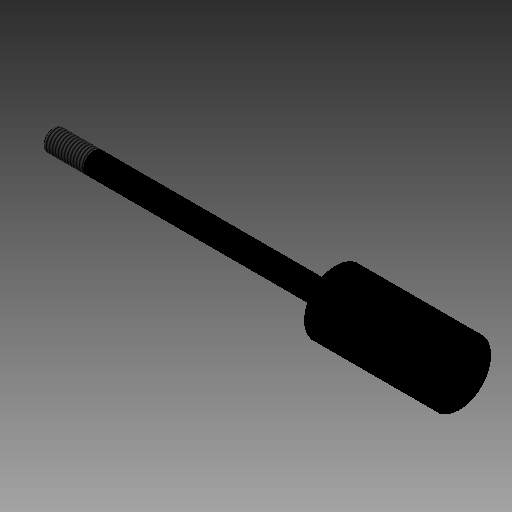
# Autodesk Inventor part: C-0420000_rod
Saved by Autodesk Inventor 2018.3 (Build 223284000, 284)
## iProperties
Category: PARTsolutions
Company: BIMBA
Created: 2019-01-30
Part Number: C-0420000_rod
Material: Generic
Catalog Web Link: www.cadenas.de
Description: Standard Air Cylinder_rod-Original Line - Standard Air Cylinders
Vendor: BIMBA
Document SubType Name: Modeling
Designer: psadmin
Manufacturer: BIMBA
Mass: 13.5965 g
Surface Area: 45.5733 cm^2
Volume: 13.5965 cm^3
Density: 1 g/cm^3
Appearance: PSOLRGB-0-0-0
PSOL_IDENT_0: {$CADENAS_DATA\23d-libs\bimba\bimba\bimba_imperial\bimba_full_line\original_line_cylinders\standard_
PSOL_IDENT_1: air_cylinders\rod.prj},319 {VTYP=3D},{NB=C-0420000_rod},{LINA=C-0420000_rod},{NN=Standard Air Cylind
PSOL_IDENT_2: er_rod},{DATE=21.03.2018 14:31:21},{GEOMDATE=09.11.2017 13:09:15},{VERSION=},{LINEID=50},{WBVAR=STRO
PSOL_IDENT_3: KE,ACTING,MNT,DER,NR,BM,CO,M,EE,EEL,K,Q,Y,F,G,T,B,H,SER,SR,NT,W,E,HL,ST,STP,PRC,PB,COLOR1,FCD,RCD,BC
PSOL_IDENT_4: D},{WBNUMERIC=STROKE,EEL,COLOR1,FCD,RCD,BCD}  {NB=C-0420000_rod},{LINA=C-0420000_rod},{KT=DUMMY},{PN=
PSOL_IDENT_5: C-042000},{DASH=},{BORE=0.75000000},{BOREPN=04},{STROKE=2.000},{STROKEALG=[0.001:50/0.001]},{STROKE1=
PSOL_IDENT_6: 2.000},{ACTING=},{ACTINGALG= '' , 'Single Acting' , 'R' , 'Reverse Single Acting' , 'D' , 'Double Ac
PSOL_IDENT_7: ting' },{ACTINGPN=},{MNT=},{MNTALG= '' , 'Front Nose Mounting' , 'P' , 'Rear Pivot Mounting' , 'BF'
PSOL_IDENT_8: , 'Front Block Mounting' , 'BR' , 'Rear Block Mounting for Vertical Positioning' , 'BFT' , 'Front Bl
PSOL_IDENT_9: ock Trunnion Mounting' , 'BRT' , 'Rear Block Trunnion Mounting' , 'A' , 'Double End Mounting with Br
PSOL_IDENT_10: ackets and Adjustable Stroke' , 'AP' , 'Rear Pivot Mounting with Adjustable Stroke' },{TYPE=C-},{MNT
PSOL_IDENT_11: PN=},{DER=},{DERALG= '' , 'N/A' },{NR=},{NRALG= '' , 'Standard' , 'NR' , 'Non-rotating - Hexagon Rod'
PSOL_IDENT_12: },{NRPN=},{BM=},{BMALG= '' , 'Without Built-in Midget 3-Way Solenoid Operated Valve' , 'LS' , 'With
PSOL_IDENT_13: Built-in Midget 3-Way Solenoid Operated Valve' },{BMPN=},{CO=},{COALG= '' , 'N/A' },{M=},{MALG= '',
PSOL_IDENT_14: 'Without Magnet', 'M', 'With Magnet' },{EE=},{EEL=0},{EEMAX=10},{EEALG= '', 'Without Extra Extensio
PSOL_IDENT_15: n', 'EE', 'With Extra Extension' },{EELALG=0},{EEPN=},{EEPN1=0.000},{K=},{KALG= '' , 'N/A' },{KPN=},
PSOL_IDENT_16: {Q=},{QALG= '' , 'Without Side Ported Rear Head' , 'Q' , 'With Side Ported Rear Head' },{QPN=},{Y=},
PSOL_IDENT_17: {YALG= '' , 'N/A' },{YPN=},{F=},{FALG= '', 'Standard', 'F', 'Molycoated Body' },{FPN=},{G=},{GPN=},{
PSOL_IDENT_18: T=},{TALG= '' , 'Standard' , 'N' , 'Low Temperature' , 'V' , 'High Temperature' },{NPN=},{VPN=},{B=}
PSOL_IDENT_19: ,{BALG= '', 'Without Bumper' , 'B' , 'With Bumper' },{BPN=},{H=},{HALG= '', 'Standard', 'H', 'With H
PSOL_IDENT_20: eavy Springs' },{HPN=},{SER=},{SERALG= '' , 'N/A' },{SR=C},{SRALG= 'C' , 'Carbon Steel Rod' , 'SR' ,
PSOL_IDENT_21: '303 Stainless Steel Rod' , '' , '303 Stainless Steel Rod1' },{SRPN=C},{SRCON=1},{NT=},{NTPN=},{W=}
PSOL_IDENT_22: ,{WALG= '' , 'N/A' },{WPN=},{E=},{EALG= '' , 'Without Special Lube and Seals' , 'E' , 'With Special
PSOL_IDENT_23: Lube and Seals' },{EPN=},{HL=},{HLALG= '' , 'N/A' },{ST=},{STALG= '' , 'Without Switch Track' , 'T'
PSOL_IDENT_24: , 'With Switch Track' },{STP=},{STPALG= '' , 'N/A' },{STPN=},{PRC=},{PRCALG= '' , 'Without Piston Ro
PSOL_IDENT_25: d Clevis' , 'D-166-1' , 'With Piston Rod Clevis' },{PRCPN=},{PB=},{PBALG= '' , 'Without Pivot Bracke
PSOL_IDENT_26: t' , 'D-167' , 'With Pivot Bracket' },{PBPN=},{TLEN=3.9460},{TEXT=0.233333},{SPACE=0.133333},{FRAC=5
PSOL_IDENT_27: .5700},{RGCON=},{RGDACCON=},{RHCON=},{RHCONON=1},{RHACCON=},{FNUTCON=1},{RNUTCON=0},{FNUTPN=D-98},{R
PSOL_IDENT_28: NUTPN=},{FNUTTRANS=0.0000},{RNUTTRANS=0.0000},{VHOLECON=2},{A1=0.8750},{A1N=0.8750},{A1P=1.5940},{A1
PSOL_IDENT_29: B=1.5940},{A4=0.3130},{A4N=0.3130},{A4P=0.2525},{A5=0.0300},{A1H=0.531},{A1NH=0.5310},{A1PH=1.5940},
PSOL_IDENT_30: {A1BH=1.0940},{A1SH=1.2190},{A2H=0.2190},{A2NH=0.2190},{LENGTH=1.5000},{LENGTH1=1.5000},{LENGTH2=3.0
PSOL_IDENT_31: 300},{MUL=3.3800},{MUL11=3.3800},{MUL22=5.3800},{MUL33=3.3800},{MUL2=1.6900},{MUL211=1.6900},{MUL222=
PSOL_IDENT_32: 2.6900},{MUL233=1.6900},{SSS=4.0000},{RGLEN=0.5920},{RHLEN=0.3420},{SSS1=3.0000},{A13=1.3120},{THDLE
PSOL_IDENT_33: N1=0.5000},{THD1=0.2500},{TAB=UNF},{THDLEN=0.5000},{THD=0.2500},{OD=0.7615},{RODL=4.8490},{PL=1.4740
PSOL_IDENT_34: },{RODDIA=0.2500},{HEX=0.2500},{RODTRANS=0.0000},{G1=0.1250},{ON=0},{G5=0.6250},{DERLEN=3.3750},{THO
PSOL_IDENT_35: LE=0.0000},{WF=0.2200},{BADD=0.0000},{MADD=0.0000},{NVADD=0.000},{JRADD=0.00000},{COLOR=0.00,0.00,0.
PSOL_IDENT_36: 00,0.00},{GROOVE=1},{HOL=0},{D7=0.2520},{H1=1.1175},{D1=0.8050},{D1RH=0.8050},{D1P=0.8325},{D1B=0.86
PSOL_IDENT_37: 25},{D1N=0.8050},{D1NRH=0.8050},{D1BRH=0.8325},{D1PRH=0.8625},{BOZO=0},{HADD=0.000},{COLOR1=0},{DEFL=
PSOL_IDENT_38: 0.0000},{HEXL=0.0000},{SSADD=0.0000},{WFL=0.0000},{MOVE=0.0000},{PRCL2=0.50000},{PRCB=0.16000},{PRCT
PSOL_IDENT_39: RANS=0.16000},{FCD=0},{RCD=0},{BCD=0}
NN: Standard Air Cylinder_rod
NT: Standard
NB: C-0420000_rod
NBSYN: $PN.$COLOR1._rod
LINA: C-0420000_rod
PN: C-042000
BORE: 0.75
BOREPN: 04
STROKE: 2
ACTING: Single Acting
MNT: Front Nose Mounting
DER: N/A
NR: Standard
BM: Without Built-in Midget 3-Way Solenoid Operated Valve
CO: N/A
M: Without Magnet
EE: Without Extra Extension
EEL: 0
K: N/A
Q: Without Side Ported Rear Head
Y: N/A
F: Standard
G: Without Magnalube Lubrication
T: Standard
B: Without Bumper
H: Standard
SER: N/A
SR: Carbon Steel Rod
W: N/A
E: Without Special Lube and Seals
HL: N/A
ST: Without Switch Track
STP: N/A
PRC: Without Piston Rod Clevis
PB: Without Pivot Bracket
A1N: 0.875
A1P: 1.594
A1B: 1.594
A4N: 0.313
A4P: 0.2525
A5: 0.03
A1NH: 0.531
A1PH: 1.594
A1BH: 1.094
A1SH: 1.219
A2NH: 0.219
A13: 1.312
THDLEN1: 0.5
THD1: 0.25
TAB: UNF
OD: 0.7615
RODDIA: 0.25
HEX: 0.25
G1: 0.125
G5: 0.625
THOLE: 0
WF: 0.22
GROOVE: 1
D7: 0.252
D1P: 0.8325
D1B: 0.8625
D1N: 0.805
D1NRH: 0.805
D1BRH: 0.8325
D1PRH: 0.8625
COLOR1: 0
FCD: 0
RCD: 0
BCD: 0
SUPPLIER: BIMBA
ARTICLENO: C-0420000_rod
BOMINFO: C-0420000_rod
CREATOR: CADENAS GmbH
Title: C-0420000_rod
Author: Cadenas PARTsolutions
Comments: Original Line - Standard Air Cylinders
Autodesk Inventor part; units mm, degrees
sketch "Sketch_1" plane through (0, 0, 0) normal (0, 0, 1) x (1, 0, 0)
  line L0 (110.4646, 0) -> (0, 0)
  line L1 (0, 0) -> (0, 3.175)
  line L2 (0, 3.175) -> (73.025, 3.175)
  line L3 (73.025, 3.175) -> (73.025, 9.6203)
  line L4 (73.025, 9.6203) -> (110.4646, 9.6203)
  line L5 (110.4646, 9.6203) -> (110.4646, 0)
  line L6 (110.4646, 0) -> (0, 0)
  constraints: 14 end point
revolve "Revolution1" add sketch "Sketch_1" angle 360 about axis through (110.4646, 0, 0) along (1, 0, 0)
sketch "Sketch_3" plane through (0, 0, 0) normal (0, 0, 1) x (1, 0, 0)
  line L0 (0, 0) -> (-12.7, 0)
  line L1 (-12.7, 0) -> (-12.7, 2.634)
  line L2 (-12.7, 2.634) -> (-12.159, 3.175)
  line L3 (-12.159, 3.175) -> (0, 3.175)
  line L4 (0, 3.175) -> (0, 0)
  line L5 (0, 0) -> (-12.7, 0)
  constraints: 12 end point
revolve "Revolution2" add sketch "Sketch_3" angle 360 about axis through (0, 0, 0) along (1, 0, 0)
thread "Thread1" size "1/4-28 UNF" class "2A" standard "ANSI Unified Screw Threads" length 12.159
sketch "Sketch_30" plane through (0, 0, 0) normal (0, 0, 1) x (1, 0, 0)
  line L0 (0, 0) -> (-0.254, 0)
  line L1 (-0.254, 2.921) -> (0, 2.921)
  line L2 (0, 2.921) -> (0, 3.429)
  line L3 (0, 3.429) -> (-0.254, 3.429)
  line L4 (-0.254, 3.429) -> (-0.254, 2.921)
  constraints: 10 end point
revolve "Revolution3" cut sketch "Sketch_30" angle 360 about axis through (0, 0, 0) along (1, 0, 0)
ref_plane "dia1_XY" through (0, 3.175, 0) normal (1, 0, 0) x (0, 0, -1)
ref_plane "dia1_YZ" through (0, 3.175, 0) normal (0, 0, -1) x (0, 1, 0)
ref_plane "dia1_ZX" through (0, 3.175, 0) normal (0, 1, 0) x (1, 0, 0)
ref_plane "dia12_XY" through (0, 0, 10.2235) normal (1, 0, 0) x (0, 0, -1)
ref_plane "dia12_YZ" through (0, 0, 10.2235) normal (0, 0, -1) x (0, 1, 0)
ref_plane "dia12_ZX" through (0, 0, 10.2235) normal (0, 1, 0) x (1, 0, 0)
ref_plane "dia2_XY" through (0, -3.175, 0) normal (1, 0, 0) x (0, 0, -1)
ref_plane "dia2_YZ" through (0, -3.175, 0) normal (0, 0, -1) x (0, 1, 0)
ref_plane "dia2_ZX" through (0, -3.175, 0) normal (0, 1, 0) x (1, 0, 0)
ref_plane "dia22_XY" through (0, 0, -10.2235) normal (1, 0, 0) x (0, 0, -1)
ref_plane "dia22_YZ" through (0, 0, -10.2235) normal (0, 0, -1) x (0, 1, 0)
ref_plane "dia22_ZX" through (0, 0, -10.2235) normal (0, 1, 0) x (1, 0, 0)
ref_plane "rl1_XY" through (-12.7, 0, 0) normal (1, 0, 0) x (0, 0, -1)
ref_plane "rl1_YZ" through (-12.7, 0, 0) normal (0, 0, -1) x (0, 1, 0)
ref_plane "rl1_ZX" through (-12.7, 0, 0) normal (0, 1, 0) x (1, 0, 0)
ref_plane "rl2_XY" through (0, 0, 0) normal (1, 0, 0) x (0, 0, -1)
ref_plane "rl2_YZ" through (0, 0, 0) normal (0, 0, -1) x (0, 1, 0)
ref_plane "rl2_ZX" through (0, 0, 0) normal (0, 1, 0) x (1, 0, 0)
ref_plane "rod_cp_XY" through (0, 0, 0) normal (1, 0, 0) x (0, 0, -1)
ref_plane "rod_cp_YZ" through (0, 0, 0) normal (0, 0, -1) x (0, 1, 0)
ref_plane "rod_cp_ZX" through (0, 0, 0) normal (0, 1, 0) x (1, 0, 0)
ref_plane "thd1_XY" through (-12.7, 3.175, 0) normal (1, 0, 0) x (0, 0, -1)
ref_plane "thd1_YZ" through (-12.7, 3.175, 0) normal (0, 0, -1) x (0, 1, 0)
ref_plane "thd1_ZX" through (-12.7, 3.175, 0) normal (0, 1, 0) x (1, 0, 0)
ref_plane "thd2_XY" through (-12.7, -3.175, 0) normal (1, 0, 0) x (0, 0, -1)
ref_plane "thd2_YZ" through (-12.7, -3.175, 0) normal (0, 0, -1) x (0, 1, 0)
ref_plane "thd2_ZX" through (-12.7, -3.175, 0) normal (0, 1, 0) x (1, 0, 0)
ref_plane "to_rod_clevis_XY" through (-16.764, 0, 0) normal (1, 0, 0) x (0, 0, -1)
ref_plane "to_rod_clevis_YZ" through (-16.764, 0, 0) normal (0, 0, -1) x (0, 1, 0)
ref_plane "to_rod_clevis_ZX" through (-16.764, 0, 0) normal (0, 1, 0) x (1, 0, 0)
body "Solid1"
